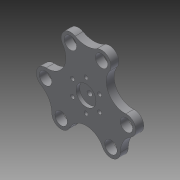
# Autodesk Inventor part: Effector_Platform
Saved by Autodesk Inventor 2014 (Build 180170000, 170)
## iProperties
Created: 2014-02-12
Part Number: Effector_Platform
Material: Generic
Document SubType Name: Modeling
Designer: ThatOtherGuy
Density: 0.952 g/cm^3
Mass: 10.8818 g
Surface Area: 65.44 cm^2
Volume: 11.4305 cm^3
Appearance: Default
Author: ThatOtherGuy
Autodesk Inventor part; units mm, degrees
note: some values were not read from the file. Chosen so that the rebuilt part matches the saved one: sketch regions of "Shape".
ref_plane "YZ Plane" through (0, 0, 0) normal (1, 0, 0) x (0, 1, 0)
ref_plane "XZ Plane" through (0, 0, 0) normal (0, 1, 0) x (-1, 0, 0)
ref_plane "XY Plane" through (0, 0, 0) normal (0, 0, 1) x (1, 0, 0)
sketch "Sketch1" plane through (0, 0, 0) normal (0, 1, 0) x (-1, 0, 0)
  circle A0 centre (0, 0) radius 2.1
  circle A1 centre (0, 0) radius 8
  circle A2 centre (0, 0) radius 12.5
  circle A3 centre (0, 0) radius 51.9615
  line L0 (-45, -25.9808) -> (-28.034, 3.4052)
  line L1 (0, 51.9615) -> (16.966, 22.5755)
  line L2 (45, -25.9808) -> (11.068, -25.9808)
  circle A4 centre (12.5, 30.3109) radius 5
  circle A5 centre (32.5, -4.3301) radius 5
  circle A6 centre (-12.5, 30.3109) radius 5
  circle A7 centre (-32.5, -4.3301) radius 5
  circle A8 centre (-20, -25.9808) radius 5
  circle A9 centre (20, -25.9808) radius 5
  circle A10 centre (0, 12.5) radius 1.6
  circle A11 centre (-10.8253, 6.25) radius 1.6
  circle A12 centre (-10.8253, -6.25) radius 1.6
  circle A13 centre (0, -12.5) radius 1.6
  circle A14 centre (10.8253, -6.25) radius 1.6
  circle A15 centre (10.8253, 6.25) radius 1.6
  circle A16 centre (-32.5, -4.3301) radius 7.5
  circle A17 centre (-12.5, 30.3109) radius 7.5
  circle A18 centre (12.5, 30.3109) radius 7.5
  circle A19 centre (32.5, -4.3301) radius 7.5
  circle A20 centre (20, -25.9808) radius 7.5
  circle A21 centre (-20, -25.9808) radius 7.5
  arc A22 (-8.75, 36.8061) -> (8.75, 36.8061) centre (0, 51.9615) ccw
  arc A23 (-27.5, -25.9808) -> (-36.25, -10.8253) centre (-45, -25.9808) ccw
  arc A24 (36.25, -10.8253) -> (27.5, -25.9808) centre (45, -25.9808) ccw
  arc A25 (13.2584, -29.2673) -> (-13.2584, -29.2673) centre (0, -35.7308) ccw
  arc A26 (-31.9754, 3.1515) -> (-18.717, 26.1158) centre (-30.9437, 17.8654) ccw
  arc A27 (18.717, 26.1158) -> (31.9754, 3.1515) centre (30.9437, 17.8654) ccw
  line L3 (-16.966, 22.5755) -> (0, 51.9615)
  line L4 (-28.034, 3.4052) -> (-16.966, 22.5755)
  line L5 (-11.068, -25.9808) -> (-45, -25.9808)
  line L6 (11.068, -25.9808) -> (-11.068, -25.9808)
  line L7 (16.966, 22.5755) -> (28.034, 3.4052)
  line L8 (28.034, 3.4052) -> (45, -25.9808)
  circle A28 centre (14.0253, 0) radius 1.6
  point P0 (-28.75, 2.1651)
  point P1 (-16.25, 23.8157)
  point P2 (16.25, 23.8157)
  point P3 (28.75, 2.1651)
  point P4 (12.5, -25.9808)
  point P5 (-12.5, -25.9808)
  dimension "d4" = 25
  dimension "d0" = 4.2
  dimension "d3" = 16
  dimension "d11" = 90
  dimension "d12" = 40
  dimension "d13" = 10
  dimension "d14" = 25
  dimension "d15" = 25
  dimension "d16" = 40
  dimension "d17" = 40
  dimension "d18" = 25
  dimension "d19" = 25
  dimension "d26" = 3.2
  dimension "d29" = 360
  dimension "d38" = 15
  dimension "d47" = 5
  dimension "d48" = 90
  dimension "d49" = 90
  dimension "d50" = 6.25
  dimension "d51" = 3.2
  constraints: 39 point on circle, 30 point on line, 28 centre point, 18 end point, 13 equal radius, 10 coincident, 9 tangent, 3 horizontal, 2 vertical alignment, 15 other
  measures "d0" diameter of A0
  measures "d3" diameter of A1
  measures "d11" distance of L1.start L2.start
  measures "d12" distance of A4.centre A5.centre
  measures "d13" diameter of A4
  measures "d14" distance of L1.start A4.centre
  measures "d15" distance of A5.centre L2.start
  measures "d16" distance of A7.centre A6.centre
  measures "d17" distance of A9.centre A8.centre
  measures "d18" distance of L0.start A8.centre
  measures "d19" distance of L0.start A7.centre
  measures "d26" diameter of A10
  measures "d38" diameter of A16
  measures "d47" distance edge to line of A25 L2
  measures "d48" distance of A23.centre L1.start
  measures "d49" distance of L2.start L0.start
  measures "d50" vertical distance of A28.centre A15.centre
  measures "d51" horizontal distance of A15.centre A28.centre
extrude "Shape" add sketch "Sketch1" along normal blind 6.731 contours A1 | A2 A28 | A2 A28 | A28 A2 A14 A13 A12 A11 A10 A15 | A15 A2 | A2 A15 | A14 A2 | A2 A14 | A10 A2 | A2 A10 | A13 A2 | A2 A13 | A11 A2 | A2 A11 | A12 A2 | A2 A12 | A18 L1 A4 | L1 A4 A18 | A18 L1 A27 L8 A19 A24 A20 L2 A25 L5 A21 A23 A16 L0 A26 L3 A17 A22 | L3 A6 A17 | A17 L3 A6 | A20 L2 A9 | L2 A9 A20 | L8 A5 A19 | A19 L8 A5 | A16 L0 A7 | L0 A7 A16 | L5 A8 A21 | A21 L5 A8 | A4 L1 | L1 A4 | A18 A27 L1 | A17 L3 A26 | L3 A6 | A6 L3 | A9 L2 | L2 A9 | A25 L2 A20 | L8 A27 A19 | L8 A5 | A5 L8 | A7 L0 | L0 A7 | A26 L0 A16 | L5 A25 A21 | L5 A8 | A8 L5
extrude "Holes" cut sketch "Sketch1" along normal up to next contours A2 A28 | A2 A28 | A15 A2 | A2 A15 | A14 A2 | A2 A14 | A10 A2 | A2 A10 | A13 A2 | A2 A13 | A11 A2 | A2 A11 | A12 A2 | A2 A12 | A4 L1 | L1 A4 | L3 A6 | A6 L3 | A9 L2 | L2 A9 | L8 A5 | A5 L8 | A7 L0 | L0 A7 | L5 A8 | A8 L5
extrude "Inset" cut sketch "Sketch1" along normal blind 3.231 contours A1
sketch "Sketch2" plane through (0, 6.731, 0) normal (0, 1, 0) x (1, 0, 0)
  circle A0 centre (-14.0253, 0) radius 1.6 projected
extrude "Extrusion7" add sketch "Sketch2" against normal up to surface (6.731 mm away)
equation "\"d14\" = d15"
equation "\"d16\" = d12"
equation "\"d17\" = d12"
equation "\"d18\" = d14"
equation "\"d19\" = d14"
equation "\"d48\" = d11"
equation "\"d49\" = d11"
equation "\"d43\" = THICKB"
equation "\"THICKA\" = 3.175"
equation "\"THICKB\" = 6.731"
equation "\"THICKC\" = 12.7"
equation "\"MAGDIA\" = 9.5"
equation "\"BALLDIA\" = 12"
body "Solid1"
